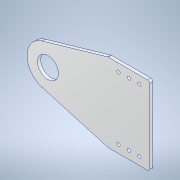
# Autodesk Inventor part: 関節3_前側板
Saved by Autodesk Inventor 2021 (Build 250183000, 183)
## iProperties
Created: 2022-02-03
Part Number: 関節3_前側板
Material: アルミニウム 6061
Document SubType Name: Modeling
Designer: hirohumi
Density: 2.7 g/cm^3
Appearance: アルミニウム - フラット
Author: hirohumi
Autodesk Inventor part; units mm, degrees
ref_plane "YZ Plane" through (0, 0, 0) normal (1, 0, 0) x (0, 1, 0)
ref_plane "XZ Plane" through (0, 0, 0) normal (0, 1, 0) x (-1, 0, 0)
ref_plane "XY Plane" through (0, 0, 0) normal (0, 0, 1) x (1, 0, 0)
sketch "スケッチ1" plane through (0, 0, 0) normal (0, 0, 1) x (1, 0, 0)
  line L0 (57.5, 37.5) -> (337.5, 37.5) construction
  line L1 (337.5, 37.5) -> (337.5, 22.5) construction
  line L2 (337.5, 22.5) -> (57.5, 22.5) construction
  line L3 (57.5, 22.5) -> (57.5, 37.5) construction
  line L4 (57.5, -37.5) -> (57.5, -22.5) construction
  line L5 (337.5, -37.5) -> (57.5, -37.5) construction
  line L6 (57.5, -22.5) -> (337.5, -22.5) construction
  line L7 (337.5, -22.5) -> (337.5, -37.5) construction
  circle A0 centre (0, 0) radius 10
  circle A1 centre (300, 0) radius 10 construction
  line L8 (330, 30) -> (270, 30) construction
  line L9 (270, 30) -> (270, -30) construction
  line L10 (270, -30) -> (330, -30) construction
  line L11 (330, -30) -> (330, 30) construction
  line L12 (330, 30) -> (270, -30) construction
  line L13 (270, 30) -> (330, -30) construction
  circle A2 centre (0, 0) radius 60 construction
  circle A3 centre (67.5, 30) radius 1.6
  circle A4 centre (77.5, 30) radius 1.6
  circle A5 centre (87.5, 30) radius 1.6
  circle A6 centre (67.5, -30) radius 1.6
  circle A7 centre (77.5, -30) radius 1.6
  circle A8 centre (87.5, -30) radius 1.6
  arc A9 (-5.5708, 19.2085) -> (-5.5708, -19.2085) centre (0, 0) ccw
  line L14 (97.5, 37.5) -> (97.5, -37.5)
  line L15 (97.5, -37.5) -> (57.5, -37.5)
  line L16 (-5.5708, -19.2085) -> (57.5, -37.5)
  line L17 (-5.5708, 19.2085) -> (57.5, 37.5)
  line L18 (57.5, 37.5) -> (97.5, 37.5)
  point P0 (300, 0)
  point P1 (57.5, 30)
  point P2 (57.5, -30)
  dimension "d0" = 15
  dimension "d1" = 280
  dimension "d2" = 15
  dimension "d3" = 280
  dimension "d4" = 20
  dimension "d5" = 20
  dimension "d6" = 60
  dimension "d7" = 60
  dimension "d8" = 7.5
  dimension "d9" = 7.5
  dimension "d10" = 7.5
  dimension "d11" = 300
  dimension "d12" = 120
  dimension "d13" = 3.2
  dimension "d14" = 3.2
  dimension "d15" = 3.2
  dimension "d16" = 10
  dimension "d17" = 10
  dimension "d18" = 10
  dimension "d19" = 3.2
  dimension "d20" = 3.2
  dimension "d21" = 3.2
  dimension "d22" = 10
  dimension "d23" = 10
  dimension "d24" = 10
  dimension "d25" = 20
  dimension "d26" = 10
  constraints: 38 end point, 10 centre point, 7 horizontal alignment, 6 parallel, 5 midpoint, 4 perpendicular, 3 coincident, 3 horizontal, 2 collinear, 2 point on circle, 2 point on line, 2 tangent, 1 vertical alignment
  measures "d0" distance of L2.end L0.start
  measures "d1" distance of L1.end L2.end
  measures "d2" distance of L5.end L6.start
  measures "d3" distance of L7.end L5.end
  measures "d4" diameter of A0
  measures "d5" diameter of A1
  measures "d6" distance of L10.end L9.end
  measures "d7" distance of L9.end L9.start
  measures "d8" distance between parallel lines of L8 L0
  measures "d9" distance between parallel lines of L5 L10
  measures "d10" distance between parallel lines of L11 L7
  measures "d11" distance of A1.centre A0.centre
  measures "d12" diameter of A2
  measures "d13" diameter of A3
  measures "d14" diameter of A4
  measures "d15" diameter of A5
  measures "d16" distance of A4.centre A3.centre
  measures "d17" distance of A5.centre A4.centre
  measures "d18" distance of A3.centre point (57.5, 30)
  measures "d19" diameter of A6
  measures "d20" diameter of A7
  measures "d21" diameter of A8
  measures "d22" distance of A7.centre A6.centre
  measures "d23" distance of A8.centre A7.centre
  measures "d24" distance of A6.centre point (57.5, -30)
  measures "d25" radius of A9
  measures "d26" distance from line of A5.centre L14
extrude "押し出し1" add sketch "スケッチ1" along normal blind 3
fillet "フィレット1" radius 2 4 edges at (57.5, 37.5, 1.5) (97.5, 37.5, 1.5) (97.5, -37.5, 1.5) (57.5, -37.5, 1.5)
equation "\"d3\" = d1"
